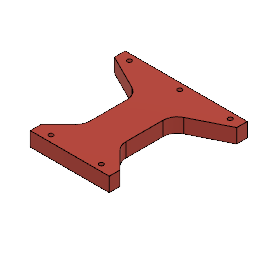
X-carriage-III-part4-rev2 v9 (Autodesk Fusion 360 design; units mm, degrees)
Autodesk Fusion 360 part; units mm, degrees
sketch "Sketch13" plane through (0, 0, 0) normal (0, 1, 0) x (1, 0, 0)
  line L0 (70, 0) -> (70, 81)
  line L1 (70, 81) -> (15, 81)
  line L2 (15, 81) -> (15, 0)
  line L3 (15, 0) -> (70, 0)
  line L4 (0, 0) -> (121.9113, 0) construction
  dimension "d66" = 55
  dimension "d130" = 81
  dimension "d131" = 15
  measures "d66" distance of L4.start
  measures "d131" distance of L4.start
extrude "Extrude10" add sketch "Sketch13" along normal blind 10
sketch "Sketch14" plane through (0, 10, 0) normal (0, 1, 0) x (-1, 0, 0)
  line L0 (-15, -81) -> (-15, 0)
  line L1 (-70, 0) -> (-70, -81)
  line L2 (-70, -81) -> (-15, -81)
  line L3 (-15, -73.5) -> (-30, -58.5)
  line L4 (-30, -58.5) -> (-30, -22.5)
  line L5 (-30, -22.5) -> (-15, -7.5)
  line L6 (-15, -40.5) -> (-70, -40.5) construction
  line L7 (-42.5, -81) -> (-42.5, 0) construction
  line L8 (-30, -40.5) -> (-87.9308, -40.5) construction
  line L9 (-70, -7.5) -> (-55, -22.5)
  line L10 (-55, -22.5) -> (-55, -58.5)
  line L11 (-55, -58.5) -> (-70, -73.5)
  circle A0 centre (-42.5, -76.5) radius 1.5
  circle A1 centre (-60, -76.5) radius 1.5
  circle A2 centre (-77.5, -76.5) radius 1.5
  circle A3 centre (-25, -76.5) radius 1.5
  circle A4 centre (-7.5, -76.5) radius 1.5
  line L12 (-7.5, -76.5) -> (-77.5, -76.5) construction
  circle A5 centre (-7.5, -4.5) radius 1.5
  circle A6 centre (-25, -4.5) radius 1.5
  circle A7 centre (-42.5, -4.5) radius 1.5
  circle A8 centre (-60, -4.5) radius 1.5
  circle A9 centre (-77.5, -4.5) radius 1.5
  line L13 (-7.5, -4.5) -> (-77.5, -4.5) construction
  line L14 (-15, 0) -> (-70, 0)
  line L15 (-30, -22.5) -> (-15, -22.5)
  line L16 (-55, -22.5) -> (-70, -22.5)
  line L17 (-30, -58.5) -> (-15, -58.5)
  line L18 (-55, -58.5) -> (-70, -58.5)
  line L19 (-70, -58.5) -> (-70, -73.5)
  line L20 (-15, -58.5) -> (-15, -73.5)
  line L21 (-15, -22.5) -> (-15, -7.5)
  line L22 (-70, -22.5) -> (-70, -7.5)
  line L23 (-70, -22.5) -> (-70, -58.5)
  line L24 (-15, -22.5) -> (-15, -58.5)
  dimension "d70" = 15
  dimension "d71" = 15
  dimension "d72" = 15
  dimension "d73" = 7.5
  dimension "d76" = 15
  dimension "d77" = 15
  dimension "d78" = 7.5
  dimension "d79" = 7.5
  dimension "d80" = 15
  dimension "d81" = 15
  dimension "d85" = 17.5
  dimension "d86" = 17.5
  dimension "d87" = 17.5
  dimension "d88" = 17.5
  dimension "d89" = 3
  dimension "d90" = 3
  dimension "d91" = 3
  dimension "d92" = 3
  dimension "d93" = 3
  dimension "d94" = 4.5
  dimension "d95" = 17.5
  dimension "d96" = 17.5
  dimension "d97" = 17.5
  dimension "d98" = 17.5
  dimension "d99" = 3
  dimension "d100" = 3
  dimension "d101" = 3
  dimension "d102" = 3
  dimension "d103" = 3
  dimension "d132" = 7.5
  dimension "d139" = 4.5
  dimension "d140" = 72
  dimension "d141" = 40.5
  measures "d70" distance of origin
  measures "d71" distance of origin
  measures "d72" distance of origin
  measures "d76" distance of origin
  measures "d77" distance of origin
  measures "d78" distance of origin
  measures "d88" distance of origin
  measures "d89" diameter of A4
  measures "d90" diameter of A3
  measures "d91" diameter of A0
  measures "d92" diameter of A1
  measures "d93" diameter of A2
  measures "d99" diameter of A5
  measures "d100" diameter of A6
  measures "d101" diameter of A7
  measures "d102" diameter of A8
  measures "d103" diameter of A9
  measures "d132" distance of origin
  measures "d139" distance of origin L13
  measures "d140" distance of L12 L13
  measures "d141" distance of origin L6
extrude "Extrude11" cut sketch "Sketch14" against normal blind 10 contours L0 L4 L15 L17 L24 | L0 L5 L15 L21 | L1 L10 L16 L18 L23 | L1 L9 L16 L22
sketch "Sketch16" plane through (0, 10, 0) normal (0, 1, 0) x (-1, 0, 0)
  line L0 (-70, -58.5) -> (-70, -81)
  line L1 (-70, -81) -> (-15, -81)
  line L2 (-15, -81) -> (-15, -58.5)
  line L3 (-30, -58.5) -> (-30, -22.5)
  circle A0 centre (-42.5, -40.5) radius 4
  line L4 (-15, 0) -> (-70, 0)
  line L5 (-70, 0) -> (-70, -7.5)
  line L6 (-55, -22.5) -> (-55, -58.5)
  line L7 (-15, -58.5) -> (-30, -58.5)
  line L8 (-30, -22.5) -> (-15, -7.5)
  line L9 (-15, -7.5) -> (-15, 0)
  line L10 (-70, -7.5) -> (-55, -22.5)
  line L11 (-55, -58.5) -> (-70, -58.5)
  dimension "d83" = 8
  measures "d83" diameter of A0
extrude "Extrude14" cut sketch "Sketch14" against normal blind 10 contours A6 | A8
sketch "Sketch17" plane through (30, 0, 0) normal (-1, 0, 0) x (0, 0, 1)
  line L0 (-58.5, 0) -> (-22.5, 0)
  line L1 (-22.5, 10) -> (-58.5, 10)
  circle A0 centre (-52.5, 6.35) radius 2
  circle A1 centre (-28.5, 6.35) radius 2
  line L2 (-52.5, 6.35) -> (-28.5, 6.35) construction
  line L3 (-58.5, 10) -> (-58.5, 0)
  line L4 (-22.5, 0) -> (-22.5, 10)
  dimension "d105" = 6.35
  dimension "d106" = 4
  dimension "d107" = 4
  dimension "d108" = 40.5
  dimension "d113" = 24
  measures "d106" diameter of A0
  measures "d107" diameter of A1
sketch "Sketch22" plane through (0, 10, 0) normal (0, 1, 0) x (-1, 0, 0)
  circle A0 centre (-60, -4.5) radius 1.5
  circle A1 centre (-25, -4.5) radius 1.5
  line L0 (-70, -58.5) -> (-70, -81)
  line L1 (-70, -81) -> (-15, -81)
  line L2 (-15, -81) -> (-15, -58.5)
  line L3 (-30, -58.5) -> (-30, -22.5)
  spline S0 degree 5 poles (-30, -22.5) (-30.6751, -22.9508) (-31.8982, -23.9212) (-33.3513, -25.5829) (-34.5873, -28.1895) (-35.2819, -31.9804) (-35.49, -36.1444) (-35.514, -40.4999) (-35.4911, -44.8557) (-35.2837, -49.0204) (-34.5894, -52.8118) (-33.353, -55.4184) (-31.8992, -57.0796) (-30.6755, -58.0495) (-30, -58.5) knots 0 0 0 0 0 0 0.1 0.2 0.3 0.4 0.5 0.6 0.7 0.8 0.9 1 1 1 1 1 1
  line L4 (-26.6736, -20.2785) -> (-33.3264, -24.7215)
  line L5 (-33.3277, -56.2805) -> (-26.6723, -60.7195)
  spline S1 degree 5 poles (-55, -22.5) (-54.3243, -22.9503) (-53.092, -23.9257) (-51.6007, -25.6127) (-50.2803, -28.2784) (-49.4997, -32.1312) (-49.3061, -36.2868) (-49.4506, -40.5251) (-49.7869, -44.6606) (-50.3396, -48.5814) (-51.2418, -52.2256) (-52.3883, -54.8952) (-53.5623, -56.7538) (-54.4956, -57.9286) (-55, -58.5) knots 0 0 0 0 0 0 0.1 0.2 0.3 0.4 0.5 0.6 0.7 0.8 0.9 1 1 1 1 1 1
  line L6 (-52.3529, -55.5012) -> (-57.6471, -61.4988)
  line L7 (-58.3285, -20.2817) -> (-51.6715, -24.7183)
  line L8 (-15, 0) -> (-70, 0)
  line L9 (-70, 0) -> (-70, -7.5)
  line L10 (-35.5, -40.5) -> (-49.5, -40.5) construction
  line L11 (-55, -22.5) -> (-55, -58.5)
  line L12 (-15, -58.5) -> (-30, -58.5)
  line L13 (-30, -22.5) -> (-15, -7.5)
  line L14 (-15, -7.5) -> (-15, 0)
  line L15 (-70, -7.5) -> (-55, -22.5)
  line L16 (-55, -58.5) -> (-70, -58.5)
  dimension "d135" = 4
  dimension "d136" = 4
  dimension "d137" = 4
  dimension "d138" = 4
  dimension "d161" = 40.5
  dimension "d162" = 14
  dimension "d163" = 35.5
extrude "Extrude22" add 1 faces at (70, 3.3333, -66) along direction (1, 0, 0) blind 15
extrude "Extrude23" add 1 faces at (15, 3.3333, -73.5) along direction (-1, 0, 0) blind 15
extrude "Extrude24" cut sketch "Sketch14" against normal through all contours A0 | A2 | A4
sketch "Sketch24" plane through (0, 0, 0) normal (0, -1, 0) x (1, 0, 0)
  circle A0 centre (7.5, -76.5) radius 1.5
  circle A1 centre (77.5, -76.5) radius 1.5
  circle A2 centre (42.5, -76.5) radius 1.5
  circle A3 centre (60, -4.5) radius 1.5
  circle A4 centre (25, -4.5) radius 1.5
  line L0 (0, -58.5) -> (0, -81)
  line L1 (0, -81) -> (85, -81)
  line L2 (85, -81) -> (85, -58.5)
  line L3 (70, -7.5) -> (70, 0)
  line L4 (70, 0) -> (15, 0)
  line L5 (15, 0) -> (15, -7.5)
  circle A5 centre (25, -4.5) radius 1.5
  circle A6 centre (60, -4.5) radius 1.5
  circle A7 centre (7.5, -76.5) radius 1.5
  circle A8 centre (42.5, -76.5) radius 1.5
  circle A9 centre (77.5, -76.5) radius 1.5
  circle A10 centre (25, -4.5) radius 3
  circle A11 centre (60, -4.5) radius 3
  circle A12 centre (7.5, -76.5) radius 3
  circle A13 centre (42.5, -76.5) radius 3
  circle A14 centre (77.5, -76.5) radius 3
  line L6 (30, -22.5) -> (30, -58.5)
  line L7 (55, -58.5) -> (55, -22.5)
  line L8 (30, -58.5) -> (0, -58.5)
  line L9 (55, -22.5) -> (70, -7.5)
  line L10 (15, -7.5) -> (30, -22.5)
  line L11 (85, -58.5) -> (55, -58.5)
  dimension "d154" = 6
  dimension "d155" = 6
  dimension "d156" = 6
  dimension "d157" = 6
  dimension "d158" = 6
  measures "d154" diameter of A10
  measures "d155" diameter of A11
  measures "d156" diameter of A12
  measures "d157" diameter of A13
  measures "d158" diameter of A14
extrude "Extrude25" cut sketch "Sketch24" against normal blind 3 contours A10 | A11 | A12 | A13 | A14
sketch "Sketch25" plane through (0, 10, 0) normal (0, 1, 0) x (-1, 0, 0)
  circle A0 centre (-7.5, -76.5) radius 1.5
  circle A1 centre (-77.5, -76.5) radius 1.5
  circle A2 centre (-42.5, -76.5) radius 1.5
  circle A3 centre (-25, -4.5) radius 1.5
  circle A4 centre (-60, -4.5) radius 1.5
  line L0 (-30, -22.5) -> (-15, -7.5)
  line L1 (-15, -7.5) -> (-15, 0)
  line L2 (-15, 0) -> (-70, 0)
  line L3 (-70, 0) -> (-70, -7.5)
  line L4 (-70, -7.5) -> (-55, -22.5)
  line L5 (-55, -22.5) -> (-55, -58.5)
  line L6 (-55, -58.5) -> (-85, -58.5)
  line L7 (-85, -58.5) -> (-85, -81)
  line L8 (-85, -81) -> (0, -81)
  line L9 (0, -81) -> (0, -58.5)
  line L10 (0, -58.5) -> (-30, -58.5)
  line L11 (-30, -58.5) -> (-30, -22.5)
  line L12 (-30, -58.5) -> (0, -73.5)
  line L13 (-55, -58.5) -> (-85, -73.5)
  line L14 (0, -73.5) -> (0, -58.5)
  line L15 (-30, -58.5) -> (0, -58.5)
  line L16 (-85, -58.5) -> (-85, -73.5)
  line L17 (-55, -58.5) -> (-85, -58.5)
  dimension "d165" = 7.5
  dimension "d166" = 7.5
extrude "Extrude26" cut sketch "Sketch25" against normal blind 10 contours L9 L10 L12 L14 L15 | L6 L7 L13 L16 L17
fillet "Fillet1" radius 10 4 edges at (30, 5, -58.5) (30, 5, -22.5) (55, 5, -58.5) (55, 5, -22.5)
equation "d105 = ( 12.7 / 2 ) * 1 mm"
equation "d108 = ( 81 / 2 ) * 1 mm"
